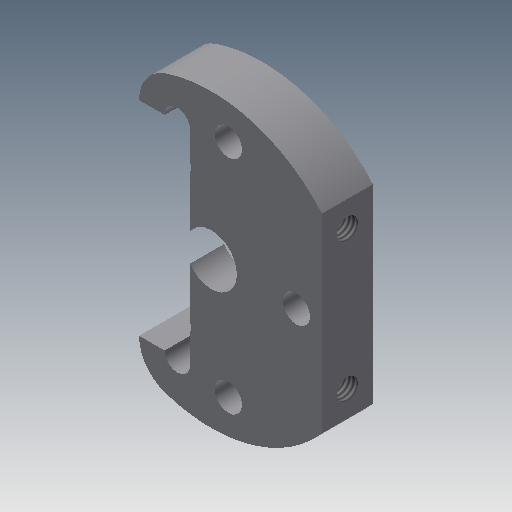
# Autodesk Inventor part: D留め板
Saved by Autodesk Inventor 2019.4 (Build 234330000, 330)
## iProperties
Created: 2018-08-09
Part Number: D留め板
Material: 一般
Document SubType Name: Modeling
Designer: Owner
Density: 1 g/cm^3
Appearance: 既定
Mass: 2.61212 g
Surface Area: 20.9911 cm^2
Volume: 2.61212 cm^3
Author: Owner
Autodesk Inventor part; units mm, degrees
ref_plane "YZ Plane" through (0, 0, 0) normal (1, 0, 0) x (0, 1, 0)
ref_plane "XZ Plane" through (0, 0, 0) normal (0, 1, 0) x (-1, 0, 0)
ref_plane "XY Plane" through (0, 0, 0) normal (0, 0, 1) x (1, 0, 0)
sketch "スケッチ1" plane through (0, 0, 0) normal (0, 0, 1) x (1, 0, 0)
  arc A0 (-2.5, -4.3301) -> (-2.5, 4.3301) centre (0, 0) ccw construction
  arc A1 (-5.423, -16.2691) -> (-5.423, 16.2691) centre (0, 0) ccw
  arc A2 (-2.5, -1.6583) -> (-2.5, 1.6583) centre (0, 0) ccw
  line L0 (-2.5, -12) -> (-2.5, -1.6583)
  line L1 (-2.5, 1.6583) -> (-2.5, 12)
  line L2 (-8.5, -12) -> (-2.5, -12)
  line L3 (-2.5, -12) -> (-2.5, 12)
  line L4 (-2.5, 12) -> (-8.5, 12)
  line L5 (-8.5, 12) -> (-8.5, -12)
  line L6 (-8.5, -12) -> (-2.5, 12) construction
  line L7 (-2.5, -12) -> (-8.5, 12) construction
  line L8 (6.2704, -6.6573) -> (-2.5, -6.6573) construction
  line L9 (-2.5, -6.6573) -> (-2.5, -9.6573) construction
  line L10 (-2.5, -9.6573) -> (6.2704, -9.6573) construction
  line L11 (6.2704, -9.6573) -> (6.2704, -6.6573) construction
  arc A3 (-5.5, -12) -> (-2.5, -12) centre (-4, -12) ccw
  arc A4 (-2.5, 12) -> (-5.5, 12) centre (-4, 12) ccw
  arc A5 (-8.5, -12) -> (-5.423, -16.2691) centre (-4, -12) ccw
  arc A6 (-5.423, 16.2691) -> (-8.5, 12) centre (-4, 12) ccw
  point P0 (-5.5, 0)
  point P1 (-5.5, 0)
  point P2 (-2.5, 13.775)
  point P3 (-2.5, -13.775)
  dimension "d0" = 10
  dimension "d2" = 6
  dimension "d9" = 2.5
  dimension "d10" = 6
  dimension "d11" = 24
  dimension "d12" = 3
  dimension "d14" = 1.5
  dimension "d15" = 3
  dimension "d16" = 3
  constraints: 24 end point, 14 point on circle, 7 centre point, 7 point on line, 5 coincident, 5 midpoint, 4 parallel, 3 tangent, 2 horizontal, 2 perpendicular, 2 vertical, 1 collinear, 1 equal radius, 1 horizontal alignment
  measures "d0" diameter of A0
  measures "d2" diameter of A2
  measures "d9" distance from line of L1 point (0, 0)
  measures "d10" distance of L1.end L4.end
  measures "d11" distance of L4.end L2.start
  measures "d12" distance of L10.end L8.start
  measures "d14" radius of A3
  measures "d15" radial gap between concentric circles of A6 A4
  measures "d16" radial gap between concentric circles of A3 A5
extrude "押し出し1" add sketch "スケッチ1" along normal blind 6 contours A5 L2 A3 L0 A2 L1 A4 L4 A6 A1
sketch "スケッチ2" plane through (0, 0, 0) normal (0, 0, -1) x (-1, 0, 0)
  circle A0 centre (0, 0) radius 5
  dimension "d6" = 10
  constraints: 1 centre point, 1 coincident
  measures "d6" diameter of A0
extrude "押し出し2" cut sketch "スケッチ2" against normal blind 2
sketch "スケッチ4" plane through (0, 0, 0) normal (0, 0, -1) x (-1, 0, 0)
  arc A0 (2.5, 4.3301) -> (2.5, -4.3301) centre (0, 0) ccw projected
  line L0 (2.5, 4.3301) -> (2.5, 12) projected
  arc A1 (5.5, 12) -> (2.5, 12) centre (4, 12) ccw projected
  line L1 (5.5, 12) -> (8.5, 12) projected
  arc A2 (8.5, 12) -> (5.423, 16.2691) centre (4, 12) ccw projected
  arc A3 (5.423, 16.2691) -> (5.423, -16.2691) centre (0, 0) ccw projected
  arc A4 (5.423, -16.2691) -> (8.5, -12) centre (4, -12) ccw projected
  line L2 (8.5, -12) -> (5.5, -12) projected
  arc A5 (2.5, -12) -> (5.5, -12) centre (4, -12) ccw projected
  line L3 (2.5, -12) -> (2.5, -4.3301) projected
  arc A6 (2.5, -7.6265) -> (2.5, -8.7036) centre (3.9, -8.1651) ccw
  arc A7 (2.5, 8.7036) -> (2.5, 7.6265) centre (3.9, 8.1651) ccw
  point P0 (2.4, 8.1651)
  point P1 (2.5, 8.1651)
  point P2 (2.4, -8.1651)
  point P3 (2.5, -8.1651)
  dimension "d17" = 1.5
  dimension "d18" = 0.1
  constraints: 6 point on circle, 4 point on line, 2 centre point, 2 horizontal alignment, 2 midpoint, 1 equal radius, 1 vertical alignment
  measures "d17" radius of A7
  measures "d18" distance of point (2.4, 8.165) point (2.5, 8.165)
extrude "押し出し3" cut sketch "スケッチ4" against normal through all contours A7 L0 | L3 A6
sketch "スケッチ5" plane through (0, 0, 0) normal (0, 0, -1) x (-1, 0, 0)
  arc A0 (2.5, -7.6265) -> (2.5, -8.7036) centre (3.9, -8.1651) ccw projected
  line L0 (2.5, -7.6265) -> (2.5, -4.3301) projected
  arc A1 (2.5, 4.3301) -> (2.5, -4.3301) centre (0, 0) ccw projected
  line L1 (2.5, 4.3301) -> (2.5, 7.6265) projected
  arc A2 (2.5, 8.7036) -> (2.5, 7.6265) centre (3.9, 8.1651) ccw projected
  line L2 (2.5, 8.7036) -> (2.5, 12) projected
  arc A3 (5.5, 12) -> (2.5, 12) centre (4, 12) ccw projected
  line L3 (5.5, 12) -> (8.5, 12) projected
  arc A4 (8.5, 12) -> (5.423, 16.2691) centre (4, 12) ccw projected
  arc A5 (5.423, 16.2691) -> (5.423, -16.2691) centre (0, 0) ccw projected
  arc A6 (5.423, -16.2691) -> (8.5, -12) centre (4, -12) ccw projected
  line L4 (8.5, -12) -> (5.5, -12) projected
  arc A7 (2.5, -12) -> (5.5, -12) centre (4, -12) ccw projected
  line L5 (2.5, -12) -> (2.5, -8.7036) projected
  line L6 (3.9, -8.1651) -> (-13, -8.1651) construction
  line L7 (3.9, 8.1651) -> (-13, 8.1651) construction
  line L8 (-13, -11.1845) -> (-13, 11.1845)
  circle A8 centre (-10, 0) radius 1.6
  circle A9 centre (-2, -13) radius 1.6
  circle A10 centre (-2, 13) radius 1.6
  line L9 (-2, -13) -> (-2, 13)
  point P0 (-2, 0)
  dimension "d21" = 13
  dimension "d22" = 3.2
  dimension "d23" = 10
  dimension "d24" = 3.2
  dimension "d25" = 3.2
  dimension "d26" = 26
  dimension "d27" = 2
  constraints: 8 end point, 3 centre point, 2 horizontal, 2 horizontal alignment, 2 point on circle, 2 point on line, 2 vertical, 1 midpoint
  measures "d21" distance from line of point (0, 0) L8
  measures "d22" diameter of A8
  measures "d23" distance of point (0, 0) A8.centre
  measures "d24" diameter of A9
  measures "d25" diameter of A10
  measures "d26" distance of L9.start L9.end
  measures "d27" distance from line of point (0, 0) L9
extrude "押し出し4" cut sketch "スケッチ5" against normal through all contours A9 | A10 | A5 L8 | A8
sketch "スケッチ6" plane through (13, -11.1845, 0) normal (1, 0, 0) x (0, 0, -1)
  line L0 (0, 3.5579) -> (0, 2.4809) projected
  line L1 (0, 19.888) -> (0, 18.811) projected
  line L2 (0, 19.3495) -> (-3, 19.3495)
  line L3 (0, 3.0194) -> (-3, 3.0194)
  point P0 (0, 11.1845)
  dimension "d30" = 3
  constraints: 4 end point, 2 horizontal, 2 midpoint, 1 vertical alignment
  measures "d30" distance of L2.start L2.end
hole "穴1" at (13, 8.1651, 3) at (13, -8.1651, 3) direction (-1, 0, 0) diameter 2.459 end through all thread size "M3x0.5" class "6H" standard "ISO Metric profile"
equation "\"d16\" = d15"
